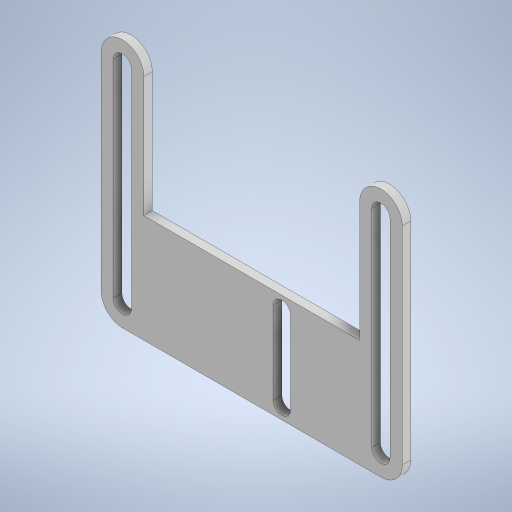
# Autodesk Inventor part: Ultrasonic Sensor
Saved by Autodesk Inventor 2024 (Build 280153000, 153)
## iProperties
Created: 2023-10-23
Part Number: Ultrasonic Sensor
Material: Generic
Document SubType Name: Modeling
Designer: olson
Density: 1 g/cm^3
Appearance: Default
Author: olson
Autodesk Inventor part; units mm, degrees
ref_plane "YZ Plane" through (0, 0, 0) normal (1, 0, 0) x (0, 1, 0)
ref_plane "XZ Plane" through (0, 0, 0) normal (0, 1, 0) x (-1, 0, 0)
ref_plane "XY Plane" through (0, 0, 0) normal (0, 0, 1) x (1, 0, 0)
sketch "Sketch1" plane through (0, 0, 0) normal (0, 0, 1) x (1, 0, 0)
  line L0 (0, -6.35) -> (25.4, -6.35)
  line L1 (25.4, -6.35) -> (25.4, -31.75)
  line L2 (25.4, -31.75) -> (-25.4, -31.75)
  line L3 (-25.4, -31.75) -> (-25.4, -6.35)
  line L4 (-25.4, -6.35) -> (0, -6.35)
  point P0 (-6.35, -6.35)
  point P1 (6.35, -6.35)
  dimension "d7" = 25.4
  dimension "d8" = 25.4
  dimension "d9" = 50.8
  constraints: 10 end point, 3 perpendicular, 3 point on line, 1 collinear, 1 horizontal
  measures "d7" distance of L0.start L0.end
  measures "d8" distance of L0.end L1.end
  measures "d9" distance of L1.end L2.end
extrude "Extrusion1" add sketch "Sketch1" along normal blind 2
sketch "Sketch2" plane through (0, 0, 2) normal (0, 0, 1) x (1, 0, 0)
  line L0 (-25.4, -6.35) -> (-25.4, -31.75) projected
  line L1 (-25.4, -31.75) -> (7.1, -31.75)
  line L2 (-25.4, -31.75) -> (25.4, -31.75) projected
  line L3 (7.1, -31.75) -> (7.1, -30.75)
  line L4 (7.1, -30.75) -> (7.1, -28.75)
  circle A0 centre (7.1, -28.75) radius 2
  circle A1 centre (7.1, -9.35) radius 2
  line L5 (5.1, -9.35) -> (5.1, -28.75)
  line L6 (9.1, -9.35) -> (9.1, -28.75)
  point P0 (0, 0)
  dimension "d10" = 32.5
  dimension "d11" = 1
  dimension "d12" = 2
  dimension "d13" = 4
  dimension "d15" = 4
  constraints: 10 end point, 4 point on circle, 4 tangent, 2 centre point, 2 point on line, 1 coincident, 1 vertical
  measures "d10" distance of L0.end L1.end
  measures "d11" distance of L1.end L3.end
  measures "d12" distance of L3.end L4.end
  measures "d13" diameter of A0
  measures "d15" diameter of A1
extrude "Extrusion2" cut sketch "Sketch2" against normal blind 2.54
sketch "Sketch3" plane through (0, 0, 0) normal (0, 0, 1) x (1, 0, 0)
  line L0 (-25.4, -6.35) -> (-25.4, -31.75) projected
  line L1 (-25.4, -6.35) -> (-25.4, -31.75)
  line L2 (-25.4, -31.75) -> (-35.4, -31.75)
  line L3 (-29.4, 26.95) -> (-35.4, 26.95)
  line L4 (-35.4, 26.95) -> (-35.4, -31.75)
  line L5 (-29.4, 26.95) -> (-25.4, 26.95)
  line L6 (-25.4, 26.95) -> (-25.4, -6.35)
  line L7 (25.4, -6.35) -> (-25.4, -6.35) projected
  line L8 (0, -6.35) -> (0, -31.75)
  line L9 (-25.4, -31.75) -> (25.4, -31.75) projected
  line L10 (25.4, -6.35) -> (25.4, -31.75)
  line L11 (25.4, -6.35) -> (25.4, -31.75)
  line L12 (25.4, -31.75) -> (35.4, -31.75)
  line L13 (29.4, 26.95) -> (35.4, 26.95)
  line L14 (35.4, 26.95) -> (35.4, -31.75)
  line L15 (29.4, 26.95) -> (25.4, 26.95)
  line L16 (25.4, 26.95) -> (25.4, -6.35)
  line L17 (-30.4, -31.75) -> (-30.4, -26.75)
  arc A0 (-32.525, -26.75) -> (-28.275, -26.75) centre (-30.4, -26.75) ccw
  line L18 (-30.4, 26.95) -> (-30.4, 21.95)
  arc A1 (-28.275, 21.95) -> (-32.525, 21.95) centre (-30.4, 21.95) ccw
  line L19 (-32.525, 21.95) -> (-32.525, -26.75)
  line L20 (-28.275, -26.75) -> (-28.275, 21.95)
  arc A2 (28.275, -26.75) -> (32.525, -26.75) centre (30.4, -26.75) ccw
  arc A3 (32.525, 21.95) -> (28.275, 21.95) centre (30.4, 21.95) ccw
  line L21 (32.525, 21.95) -> (32.525, -26.75)
  line L22 (28.275, -26.75) -> (28.275, 21.95)
  point P0 (0, 0)
  dimension "d26" = 10
  dimension "d36" = 5
  dimension "d37" = 4.25
  dimension "d38" = 5
  dimension "d39" = 4.25
  constraints: 40 end point, 10 symmetric about line, 8 point on circle, 4 centre point, 3 midpoint, 3 point on line, 3 tangent, 3 vertical, 2 coincident, 2 horizontal, 2 perpendicular, 2 other
  measures "d26" distance of L0.end L2.end
  measures "d36" distance of L17.start L17.end
  measures "d37" diameter of A0
  measures "d38" distance of L18.start L18.end
  measures "d39" diameter of A1
extrude "Extrusion3" add sketch "Sketch3" along normal blind 2 contours L0 L2 L17 A0 L20 A1 L18 L3 L5 L6 | L2 L4 L3 L18 A1 L19 A0 L17 | L16 L15 L13 L14 L12 L10
fillet "Fillet1" radius 5 6 edges at (-35.4, 26.95, 1) (-25.4, 26.95, 1) (-35.4, -31.75, 1) (25.4, 26.95, 1) (35.4, 26.95, 1) (35.4, -31.75, 1)
body "Solid1"
